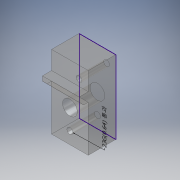
# Autodesk Inventor part: Top
Saved by Autodesk Inventor 2019 (Build 230136000, 136)
## iProperties
Created: 2019-02-07
Part Number: Top
Material: 유리
Document SubType Name: Modeling
Designer: Jeong Ji Hoon
Density: 2.18 g/cm^3
Appearance: 연회색 반사
Author: Jeong Ji Hoon
## iProperties of the stored document Top_3D 인쇄.ipt
Created: 2019-02-27
Part Number: Top_3D 인쇄
Material: 일반
Document SubType Name: Modeling
Designer: Jeong Ji Hoon
Density: 1 g/cm^3
Appearance: 기본값
Author: Jeong Ji Hoon
Autodesk Inventor part; units mm, degrees
ref_plane "YZ Plane" through (0, 0, 0) normal (1, 0, 0) x (0, 1, 0)
ref_plane "XZ Plane" through (0, 0, 0) normal (0, 1, 0) x (-1, 0, 0)
ref_plane "XY Plane" through (0, 0, 0) normal (0, 0, 1) x (1, 0, 0)
sketch "스케치1" plane through (0, 0, 0) normal (0, 0, 1) x (1, 0, 0)
  line L0 (0, 0) -> (4, 0)
  line L1 (4, 0) -> (4, 8)
  line L2 (4, 8) -> (0, 8)
  line L3 (0, 8) -> (0, 0)
  dimension "d0" = 4
  dimension "d1" = 8
  constraints: 8 end point, 2 parallel, 1 horizontal, 1 perpendicular
  measures "d0" distance of L2.end L1.end
  measures "d1" distance of L1.end L0.end
extrude "돌출1" add sketch "스케치1" along normal blind 3
sketch "스케치2" plane through (0, 0, 3) normal (0, 0, 1) x (1, 0, 0)
  line L0 (4, 8) -> (0, 8) construction
  line L1 (2, 8) -> (2, 0) construction
  line L2 (0, 0) -> (4, 0) construction
  line L3 (0, 6) -> (4, 6)
  line L4 (4, 6) -> (4, 5)
  line L5 (4, 5) -> (0, 5)
  line L6 (0, 5) -> (0, 6)
  line L7 (4, 0) -> (4, 8) projected
  line L8 (0, 8) -> (0, 0) projected
  point P0 (2, 6.7)
  point P1 (2, 3.5)
  point P2 (2, 1.3)
  point P3 (3, 6.7)
  dimension "d7" = 1
  dimension "d8" = 2
  dimension "d9" = 1.3
  dimension "d45" = 1.3
  dimension "d51" = 3.2
  dimension "d52" = 2.2
  dimension "d53" = 1
  constraints: 10 end point, 3 point on line, 2 collinear, 2 midpoint, 2 parallel, 1 horizontal, 1 horizontal alignment, 1 perpendicular
  measures "d7" distance between parallel lines of L5 L3
  measures "d8" distance between parallel lines of L0 L3
  measures "d9" distance from line of L0 point (2, 6.7)
  measures "d45" distance from line of point (2, 1.3) L2
  measures "d51" distance of point (2, 3.5) point (2, 6.7)
  measures "d52" distance of point (2, 1.3) point (2, 3.5)
  measures "d53" distance of point (3, 6.7) point (2, 6.7)
extrude "돌출2" add sketch "스케치2" along normal blind 1
hole "구멍1" at (3, 6.7, 3) direction (0, 0, -1) diameter 0.63 end through all
hole "구멍2" at (2, 3.5, 3) direction (0, 0, -1) diameter 1.6 end through all
hole "구멍3" at (2, 1.3, 3) direction (0, 0, -1) diameter 0.65 end through all
chamfer "모따기1" distance 0.5 angle 45 1 edges at (2, 5, 4)
equation "\"G23_M\" = 0.67"
equation "\"G23_F\" = 0.65"
